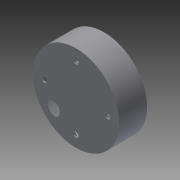
# Autodesk Inventor part: obudowa - czujnik czadu - dol v2
Saved by Autodesk Inventor 2014 (Build 180170000, 170)
## iProperties
Created: 2018-02-27
Part Number: obudowa - czujnik czadu - dol v2
Material: Generic
Document SubType Name: Modeling
Designer: HP820
Density: 1 g/cm^3
Appearance: Default
Author: HP820
Autodesk Inventor part; units mm, degrees
ref_plane "YZ Plane" through (0, 0, 0) normal (1, 0, 0) x (0, 1, 0)
ref_plane "XZ Plane" through (0, 0, 0) normal (0, 1, 0) x (-1, 0, 0)
sketch "Sketch1" plane through (0, 0, 0) normal (0, 1, 0) x (-1, 0, 0)
  circle A0 centre (0, 0) radius 34
  dimension "d0" = 68
  constraints: 1 centre point, 1 coincident
  measures "d0" diameter of A0
extrude "Extrusion1" add sketch "Sketch1" along normal blind 3
sketch "Sketch2" plane through (0, 3, 0) normal (0, 1, 0) x (1, 0, 0)
  circle A0 centre (0, 0) radius 34 projected
  circle A1 centre (0, 0) radius 31
  dimension "d3" = 62
  constraints: 1 centre point, 1 coincident
  measures "d3" diameter of A1
extrude "Extrusion2" add sketch "Sketch2" along normal blind 19
sketch "Sketch3" plane through (0, 3, 0) normal (0, 1, 0) x (1, 0, 0)
  circle A0 centre (0, 0) radius 31 projected
  circle A1 centre (0, 25) radius 2
  circle A2 centre (0, -25) radius 2
  circle A3 centre (-25, 0) radius 2
  circle A4 centre (25, 0) radius 2
  circle A5 centre (0, 0) radius 31 projected
  dimension "d6" = 4
  dimension "d7" = 4
  dimension "d8" = 4
  dimension "d9" = 4
  dimension "d10" = 25
  dimension "d11" = 25
  dimension "d12" = 25
  dimension "d13" = 25
  constraints: 4 centre point
  measures "d6" diameter of A1
  measures "d7" diameter of A2
  measures "d8" diameter of A3
  measures "d9" diameter of A4
  measures "d10" distance of A0.centre A3.centre
  measures "d11" distance of A0.centre A4.centre
  measures "d12" distance of A0.centre A2.centre
  measures "d13" distance of A1.centre A0.centre
extrude "Extrusion3" cut sketch "Sketch3" against normal up to next contours A1 | A2 | A3 | A4
chamfer "Chamfer1" distance 2 angle 45 4 edges at (-27, 3, 0) (-2, 3, 25) (23, 3, 0) (-2, 3, -25)
sketch "Sketch4" plane through (0, 3, 0) normal (0, 1, 0) x (1, 0, 0)
  circle A0 centre (-17.7645, 16.1003) radius 5
  dimension "d19" = 10
  constraints: 1 centre point
  measures "d19" diameter of A0
extrude "Extrusion4" cut sketch "Sketch4" against normal up to next
chamfer "Chamfer2" distance 3 angle 45 1 edges at (-22.7645, 3, -16.1003)
sketch "Sketch5" plane through (0, 3, 0) normal (0, 1, 0) x (1, 0, 0)
  arc A0 (-25.6588, 17.3961) -> (-19.8281, 23.8295) centre (-17.7645, 16.1003) ccw projected
  arc A1 (-25.6588, 17.3961) -> (-19.8281, 23.8295) centre (0, 0) ccw projected
  circle A2 centre (25, 0) radius 4 projected
  circle A3 centre (-25, 0) radius 4 projected
  circle A4 centre (0, -25) radius 4 projected
  circle A5 centre (0, 25) radius 4 projected
  line L0 (-7.1977, 20) -> (17.8023, 20)
  line L1 (17.8023, 20) -> (17.8023, -20)
  line L2 (17.8023, -20) -> (-7.1977, -20)
  line L3 (-7.1977, -20) -> (-7.1977, 20)
  line L4 (-12.5, 20) -> (12.5, -20) construction
  line L5 (12.5, 20) -> (-12.5, -20) construction
  dimension "d25" = 25
  dimension "d26" = 40
  constraints: 12 end point, 2 midpoint, 2 parallel, 1 horizontal, 1 perpendicular
  measures "d25" distance of L1.end L2.end
  measures "d26" distance of L0.end L1.end
sketch "Sketch6" plane through (0, 3, 0) normal (0, 1, 0) x (1, 0, 0)
  circle A0 centre (-4.1956, 16.9861) radius 1.25
  circle A1 centre (-4.1956, 16.9861) radius 3
  circle A2 centre (14.8044, 16.9861) radius 1.25
  circle A3 centre (14.8044, 16.9861) radius 3
  circle A4 centre (-4.1956, -17.0139) radius 1.25
  circle A5 centre (-4.1956, -17.0139) radius 3
  circle A6 centre (14.8044, -17.0139) radius 1.25
  circle A7 centre (14.8044, -17.0139) radius 3
  line L0 (-7.1956, 19.9861) -> (17.8044, 19.9861)
  line L1 (17.8044, 19.9861) -> (17.8044, -20.0139)
  line L2 (17.8044, -20.0139) -> (-7.1956, -20.0139)
  line L3 (-7.1956, -20.0139) -> (-7.1956, 19.9861)
  dimension "d27" = 2.5
  dimension "d28" = 6
  dimension "d29" = 2.5
  dimension "d30" = 6
  dimension "d31" = 2.5
  dimension "d32" = 6
  dimension "d33" = 2.5
  dimension "d34" = 6
  dimension "d35" = 25
  dimension "d36" = 40
  dimension "d37" = 3
  dimension "d38" = 3
  dimension "d39" = 3
  dimension "d40" = 3
  dimension "d41" = 3
  dimension "d42" = 3
  dimension "d43" = 3
  dimension "d44" = 3
  constraints: 8 centre point, 8 end point, 4 coincident, 2 parallel, 1 horizontal, 1 perpendicular
  measures "d27" diameter of A0
  measures "d28" diameter of A1
  measures "d29" diameter of A2
  measures "d30" diameter of A3
  measures "d31" diameter of A4
  measures "d32" diameter of A5
  measures "d33" diameter of A6
  measures "d34" diameter of A7
  measures "d35" distance of L1.end L2.end
  measures "d36" distance of L0.end L1.end
  measures "d37" distance from line of L3 A1.centre
  measures "d38" distance from line of L0 A0.centre
  measures "d39" distance from line of L1 A2.centre
  measures "d40" distance from line of L0 A2.centre
  measures "d41" distance from line of L2 A7.centre
  measures "d42" distance from line of L1 A6.centre
  measures "d43" distance from line of L3 A4.centre
  measures "d44" distance from line of L2 A4.centre
extrude "Extrusion5" add sketch "Sketch6" along normal blind 3 contours A1 | A3 | A5 | A7
sketch "Sketch7" plane through (-4.1956, 3, 17.0139) normal (0, 1, 0) x (1, 0, 0)
  circle A0 centre (0, 0) radius 1.25 projected
  circle A1 centre (19, 0) radius 1.25 projected
  circle A2 centre (19, 0) radius 3 projected
  circle A3 centre (0, 34) radius 1.25 projected
  circle A4 centre (0, 34) radius 3 projected
  circle A5 centre (19, 34) radius 1.25 projected
  circle A6 centre (19, 34) radius 3 projected
  point P0 (4.1956, 17.0139)
extrude "Extrusion6" cut sketch "Sketch7" against normal blind 2 contours A0 | A1 | A3 | A5
chamfer "Chamfer3" distance 0.6 angle 45 4 edges at (-5.4456, 6, 17.0139) (13.5544, 6, 17.0139) (13.5544, 6, -16.9861) (-5.4456, 6, -16.9861)
ref_plane "Work Plane1" through (13.0817, 17, 36.7639) normal (0, 0, -1) x (-1, 0, 0)
sketch "Sketch10" plane through (0, 22, 0) normal (0, 1, 0) x (1, 0, 0)
  circle A0 centre (0, 0) radius 31 projected
  arc A1 (-28.3225, 12.603) -> (-19.5355, 24.07) centre (-27.5695, 21.1262) ccw
  arc A2 (27.8015, -13.7141) -> (20.2887, -23.4387) centre (26.2341, -20.2675) ccw
  constraints: 8 point on circle, 2 centre point
extrude "Extrusion9" add sketch "Sketch10" against normal blind 6 contours A1 A0 | A0 A2
chamfer "Chamfer5" distance 4 angle 45 2 edges at (-20.7779, 16, -15.9218) (20.9018, 16, 16.1479)
sketch "Sketch11" plane through (0, 22, 0) normal (0, 1, 0) x (1, 0, 0)
  circle A0 centre (0, 0) radius 34 projected
  circle A1 centre (0, 0) radius 29.5
  line L0 (-23.6117, 17.6844) -> (23.6431, -17.6424)
  circle A2 centre (-23.6117, 17.6844) radius 1
  circle A3 centre (23.6431, -17.6424) radius 1
  dimension "d67" = 59
  dimension "d68" = 2
  dimension "d69" = 2
  constraints: 3 centre point, 3 coincident, 2 end point, 2 point on circle
  measures "d67" diameter of A1
  measures "d68" diameter of A2
  measures "d69" diameter of A3
extrude "Extrusion10" cut sketch "Sketch11" against normal blind 6 contours A2 L0 A1 | A1 A2 | A3 A1 | A1 L0 A3 | L0 A2 A1 | A1 A3 L0
chamfer "Chamfer6" distance 0.5 angle 45 2 edges at (22.6431, 22, 17.6424) (-24.6117, 22, -17.6844)
equation "\"d11\" = d10"
equation "\"d12\" = d10"
equation "\"d13\" = d10"
body "Solid1"
